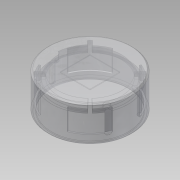
# Autodesk Inventor part: top_big_touch
Saved by Autodesk Inventor 2015 SP2 (Build 190223200, 223)
## iProperties
Created: 2015-01-05
Part Number: top_big_touch
Material: Acrylic
Document SubType Name: Modeling
Designer: Mathieu
Density: 1.188 g/cm^3
Appearance: Transparent - Clear
Mass: 2.31975 g
Surface Area: 31.9125 cm^2
Volume: 1.95266 cm^3
Author: Mathieu
Autodesk Inventor part; units mm, degrees
ref_plane "YZ Plane" through (0, 0, 0) normal (1, 0, 0) x (0, 1, 0)
ref_plane "XZ Plane" through (0, 0, 0) normal (0, 1, 0) x (-1, 0, 0)
ref_plane "XY Plane" through (0, 0, 0) normal (0, 0, 1) x (1, 0, 0)
sketch "Sketch2" plane through (0, 0, 0) normal (0, 1, 0) x (-1, 0, 0)
  line L0 (0, -1) -> (-10.5, -1)
  line L1 (-14, 0) -> (0, 0)
  line L2 (0, 0) -> (0, -1)
  line L3 (-12.75, -12) -> (-14, -12)
  line L4 (-14, 0) -> (-14, -12)
  line L5 (0, -7.6913) -> (0, 5.6913)
  line L6 (-12.75, -3.75) -> (-12.75, -12)
  line L7 (-10.5, -1) -> (-10.5, -2.5)
  line L8 (-10.5, -2.5) -> (-11.5, -2.5)
  line L9 (-11.5, -2.5) -> (-11.5, -3.75)
  line L10 (-11.5, -3.75) -> (-12.75, -3.75)
  dimension "d3" = 12
  dimension "d5" = 28
  dimension "d113" = 1
  dimension "d119" = 1.5
  dimension "d120" = 1.25
  dimension "d140" = 21
  dimension "d141" = 23
  dimension "d152" = 1.25
  dimension "d155" = 25.5
  constraints: 22 end point, 3 horizontal, 3 vertical, 1 collinear, 1 midpoint, 1 parallel, 1 perpendicular, 1 point on line
  measures "d3" distance of L1.start L3.end
  measures "d5" diameter of L4 L5
  measures "d113" distance of L1.end L0.start
  measures "d119" distance between parallel lines of L8 L0
  measures "d120" distance between parallel lines of L8 L10
  measures "d140" diameter of L7 L5
  measures "d141" diameter of L9 L5
  measures "d152" distance between parallel lines of L4 L6
  measures "d155" diameter of L6 L5
revolve "Revolution1" add sketch "Sketch2" angle 360 about axis through (0, 0, -7.6913) along (0, 0, 1)
ref_plane "Work Plane3" through (0, 0, -2) normal (0, 0, -1) x (-1, 0, 0)
chamfer "Chamfer1" distance 0.5 angle 45 2 edges at (-14, 0, 0) (-14, 0, -12)
sketch "Sketch7" plane through (0, 0, -1) normal (0, 0, -1) x (-1, 0, 0)
  line L0 (-5, -5) -> (-5, 5)
  line L1 (-5, 5) -> (5, 5)
  line L2 (5, 5) -> (5, -5)
  line L3 (5, -5) -> (-5, 5) construction
  line L4 (-5, -5) -> (5, 5) construction
  line L5 (5, -5) -> (-5, -5)
  circle A0 centre (0, 0) radius 10.5 projected
  circle A1 centre (0, 0) radius 10.5 construction
  point P0 (0, 0)
  dimension "d35" = 10
  dimension "d36" = 10
  constraints: 12 end point, 4 midpoint, 2 coincident, 2 parallel, 1 horizontal, 1 perpendicular
  measures "d35" distance of L1.end L2.end
  measures "d36" distance of L0.end L1.end
extrude "Extrusion3" cut sketch "Sketch7" against normal blind 0.25 contours L0 L1 L2 L5
sketch "Sketch3" plane through (0, 0, -2) normal (0, 0, -1) x (-1, 0, 0)
  circle A0 centre (0, 0) radius 11.5
  circle A1 centre (0, 0) radius 11.5 construction
  line L0 (0, 11.5) -> (0, -11.5) construction
  line L1 (4.8601, -10.4225) -> (-4.8601, 10.4225) construction
  line L2 (4.8601, 10.4225) -> (-4.8601, -10.4225) construction
  arc A2 (-0.8993, 11.4648) -> (0.8993, 11.4648) centre (0, 11.5) ccw
  arc A3 (5.6603, -10.0106) -> (4.0302, -10.7707) centre (4.8601, -10.4225) ccw
  arc A4 (-4.0302, -10.7707) -> (-5.6603, -10.0106) centre (-4.8601, -10.4225) ccw
  arc A5 (-5.6603, -10.0106) -> (-4.0302, -10.7707) centre (0, 0) ccw
  arc A6 (4.0302, -10.7707) -> (5.6603, -10.0106) centre (0, 0) ccw
  arc A7 (0.8993, 11.4648) -> (-0.8993, 11.4648) centre (0, 0) ccw
  circle A8 centre (0, 0) radius 14 projected
  circle A9 centre (0, 0) radius 11.5 projected
  dimension "d17" = 25
  dimension "d18" = 25
  dimension "d33" = 1.8
  constraints: 19 point on circle, 7 centre point, 6 end point, 4 coincident, 4 midpoint, 2 equal radius, 1 vertical, 1 vertical alignment, 16 other
  measures "d17" angle of L0 L2
  measures "d18" angle of L1 L0
  measures "d33" diameter of A2
extrude "Extrusion1" add sketch "Sketch3" along normal up to surface (1.75 mm away) contours A2 A0 | A0 A3 | A4 A0
sketch "Sketch16" plane through (0, 0, -3.75) normal (0, 0, -1) x (-1, 0, 0)
  line L0 (0, 0) -> (5.3884, -11.5554) construction
  line L1 (0, 0) -> (-5.3884, -11.5554) construction
  line L2 (0, 0) -> (0, 12.75) construction
  circle A0 centre (-5.3884, -11.5554) radius 0.9
  circle A1 centre (5.3884, -11.5554) radius 0.9
  circle A2 centre (0, 12.75) radius 0.9
  circle A3 centre (0, 0) radius 12.75 projected
  point P0 (0, 0)
  dimension "d121" = 25
  dimension "d122" = 25
  dimension "d148" = 1.8
  constraints: 6 end point, 3 centre point, 3 coincident, 3 point on circle, 2 equal radius, 1 vertical
  measures "d121" angle of L2 L1
  measures "d122" angle of L2 L0
  measures "d148" diameter of A0
extrude "Extrusion6" add sketch "Sketch16" along normal blind 6.75 contours A0 A3 | A3 A0 | A3 A2 | A2 A3 | A3 A1 | A1 A3
ref_plane "Work Plane1" through (0, 0, -1.1768) normal (0.7071068, 0.7071068, 0) x (0, 0, 1)
sketch "Sketch9" plane through (0, 0, -1.1768) normal (0.7071068, 0.7071068, 0) x (0, 0, 1)
  line L0 (-8.3232, -13.25) -> (-1.3232, -13.25)
  line L1 (-1.3232, -13.25) -> (-1.3232, -12.75)
  line L2 (-1.3232, -12.75) -> (-8.3232, -12.75)
  line L3 (-8.3232, -12.75) -> (-8.3232, -13.25)
  line L4 (-8.3232, -13.25) -> (-1.3232, -12.75) construction
  line L5 (-1.3232, -13.25) -> (-8.3232, -12.75) construction
  line L6 (1.1768, 13.5) -> (1.1768, -13.5) projected
  line L7 (3.5768, 0) -> (-13.2232, 0) projected
  line L8 (-9.3232, -9.6292) -> (-2.5732, -9.6292) projected
  line L9 (-2.5732, 3.5047) -> (-2.5732, -9.6292) projected
  line L10 (-2.5732, 3.5047) -> (-9.3232, 3.5047) projected
  line L11 (-9.3232, 3.5047) -> (-9.3232, 5.1951) projected
  line L12 (-9.3232, 5.1951) -> (-2.5732, 5.1951) projected
  line L13 (-2.5732, 11.6436) -> (-2.5732, 5.1951) projected
  line L14 (-2.5732, 11.6436) -> (-9.3232, 11.6436) projected
  line L15 (-9.3232, 11.6436) -> (-9.3232, 12.2589) projected
  line L16 (-9.3232, 12.2589) -> (-2.5732, 12.2589) projected
  line L17 (-2.5732, -8.3572) -> (-2.5732, 12.2589) projected
  line L18 (-2.5732, -8.3572) -> (-9.3232, -8.3572) projected
  line L19 (-9.3232, -8.3572) -> (-9.3232, -9.6292) projected
  line L20 (-10.8232, 12.75) -> (-10.8232, -12.75) projected
  line L21 (-2.5732, 3.5047) -> (-2.5732, -12.75) projected
  point P0 (1.1768, 0)
  point P1 (-4.8232, -13)
  dimension "d59" = 0.5
  dimension "d60" = 7
  dimension "d153" = 12.75
  dimension "d154" = 12.75
  dimension "d161" = 12
  dimension "d162" = 6
  constraints: 12 end point, 2 midpoint, 2 parallel, 1 horizontal, 1 perpendicular
  measures "d59" distance of L0.end L1.end
  measures "d60" distance of L0.start L0.end
  measures "d153" distance from line of L20.end L7
  measures "d154" distance between parallel lines of L7 L2
  measures "d161" distance between parallel lines of L6 L20
  measures "d162" distance from line of L6 point (-4.823, -13)
revolve "Revolution2" cut sketch "Sketch9" angle 48 mid plane about axis through (0, 0, -11.5) along (0, 0, -1) contours L3 L2 L1 L0
pattern_circular "Circular Pattern1" count 4 over 360 about axis through (0, 0, -11.5) along (0, 0, -1) of "Revolution2"
sketch "Sketch17" plane through (0, 0, -3.75) normal (0, 0, -1) x (-1, 0, 0)
  line L0 (7.0937, 7.7414) -> (8.9516, 9.7689)
  line L1 (7.7414, 7.0937) -> (9.7689, 8.9516)
  line L2 (0, 0) -> (9.0478, 9.0478) construction
  arc A0 (9.7689, 8.9516) -> (8.9516, 9.7689) centre (0, 0) ccw
  circle A1 centre (0, 0) radius 10.5 projected
  line L3 (-19.6, -19.6) -> (19.6, 19.6) construction
  line L4 (12.3699, 4.7484) -> (0, 0) construction
  line L5 (11.9032, 4.5692) -> (12.3699, 4.7484) projected
  line L6 (0, 0) -> (4.7484, 12.3699) construction
  arc A2 (12.3699, 4.7484) -> (4.7484, 12.3699) centre (0, 0) ccw projected
  arc A3 (7.7414, 7.0937) -> (7.0937, 7.7414) centre (0, 0) ccw
  point P0 (0.8993, 11.4648)
  point P1 (0, 0)
  dimension "d128" = 2.5
  dimension "d129" = 5
  dimension "d160" = 48
  constraints: 10 end point, 4 point on circle, 2 centre point, 2 coincident, 2 collinear, 2 point on line, 1 concentric, 3 other
  measures "d128" angle of L2 L1
  measures "d129" angle of L0 L1
  measures "d160" angle of L4 L6
extrude "Extrusion7" cut sketch "Sketch17" against normal up to surface (2.75 mm away) contours L0 A0 L1 A1
pattern_circular "Circular Pattern3" count 4 over 360 about axis through (0, 0, -11.5) along (0, 0, -1) of "Extrusion7"
chamfer "Chamfer2" distance 0.125 distance2 0.25 1 edges at (-12.75, 0, -12) measured on face at (-13.25, 0, -12)
sketch "Sketch19" plane through (0, 0, -2.5) normal (0, 0, -1) x (-1, 0, 0)
  arc A0 (7.0937, 7.7414) -> (-7.0937, 7.7414) centre (0, 0) ccw projected
  arc A1 (5.6603, -10.0106) -> (4.0302, -10.7707) centre (4.8601, -10.4225) ccw projected
  arc A2 (5.6603, -10.0106) -> (7.7693, -8.4787) centre (0, 0) ccw projected
  arc A3 (8.4787, -7.7693) -> (8.4787, 7.7693) centre (0, 0) ccw projected
  arc A4 (7.7693, 8.4787) -> (0.8993, 11.4648) centre (0, 0) ccw projected
  arc A5 (-0.8993, 11.4648) -> (0.8993, 11.4648) centre (0, 11.5) ccw projected
  arc A6 (-0.8993, 11.4648) -> (-7.7693, 8.4787) centre (0, 0) ccw projected
  arc A7 (-8.4787, 7.7693) -> (-8.4787, -7.7693) centre (0, 0) ccw projected
  arc A8 (-7.7693, -8.4787) -> (-5.6603, -10.0106) centre (0, 0) ccw projected
  arc A9 (-4.0302, -10.7707) -> (-5.6603, -10.0106) centre (-4.8601, -10.4225) ccw projected
  arc A10 (-4.0302, -10.7707) -> (4.0302, -10.7707) centre (0, 0) ccw projected
  line L0 (-7.7693, 8.4787) -> (-7.0937, 7.7414) projected
  line L1 (7.0937, 7.7414) -> (7.7693, 8.4787) projected
  line L2 (7.7414, -7.0937) -> (8.4787, -7.7693) projected
  line L3 (8.4787, 7.7693) -> (7.7414, 7.0937) projected
  arc A11 (7.7414, -7.0937) -> (7.7414, 7.0937) centre (0, 0) ccw projected
  line L4 (-8.4787, -7.7693) -> (-7.7414, -7.0937) projected
  arc A12 (-7.7414, 7.0937) -> (-7.7414, -7.0937) centre (0, 0) ccw projected
  line L5 (-7.7414, 7.0937) -> (-8.4787, 7.7693) projected
  line L6 (7.7693, -8.4787) -> (7.0937, -7.7414) projected
  arc A13 (-7.0937, -7.7414) -> (7.0937, -7.7414) centre (0, 0) ccw projected
  line L7 (-7.0937, -7.7414) -> (-7.7693, -8.4787) projected
  line L8 (0, 0) -> (0, 10.6)
  line L9 (0, 0) -> (-7.7693, 8.4787)
  constraints: 9 end point, 4 point on circle, 1 vertical
extrude "Extrusion10" cut sketch "Sketch19" against normal up to surface (1.5 mm away) contours L8 L9 A0 | A0 L0 A6 A5 L8
chamfer "Chamfer3" distance 0.5 angle 45 3 edges at (0, 11.85, -10.5) (5.008, -10.7397, -10.5) (-5.008, -10.7397, -10.5)
chamfer "Chamfer4" distance 0.5 angle 45 10 edges at (4.4798, -9.6069, -3.75) (6.7583, -9.3046, -3.75) (0, -11.5, -3.75) (11.5, 0, -3.75) (-4.4798, -9.6069, -3.75) (-6.7583, -9.3046, -3.75) (-11.5, 0, -3.75) (-4.5842, 10.5468, -3.75) (0, 10.6, -3.75) (4.5842, 10.5468, -3.75)
body "Solid1"
